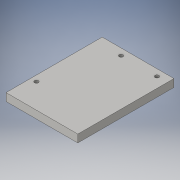
# Autodesk Inventor part: Arduino
Saved by Autodesk Inventor 2016 (Build 200138000, 138)
## iProperties
Created: 2018-09-29
Part Number: Arduino
Material: Generic
Document SubType Name: Modeling
Designer: Kyle
Density: 1 g/cm^3
Appearance: Default
Author: Kyle
## iProperties of the stored document Arduino_3DPrint.ipt
Created: 2018-09-30
Part Number: Arduino_3DPrint
Material: Generic
Document SubType Name: Modeling
Designer: Kyle
Density: 1 g/cm^3
Appearance: Default
Author: Kyle
Autodesk Inventor part; units mm, degrees
ref_plane "YZ Plane" through (0, 0, 0) normal (1, 0, 0) x (0, 1, 0)
ref_plane "XZ Plane" through (0, 0, 0) normal (0, 1, 0) x (-1, 0, 0)
ref_plane "XY Plane" through (0, 0, 0) normal (0, 0, 1) x (1, 0, 0)
sketch "Sketch1" plane through (0, 0, 0) normal (0, 1, 0) x (-1, 0, 0)
  circle A0 centre (24, 19) radius 1.5
  circle A1 centre (-19.5, -31.5) radius 1.5
  circle A2 centre (-19.5, -31.5) radius 1.5
  circle A3 centre (8.5, -31.5) radius 1.5
  line L0 (0, 0) -> (0, 17.5)
  line L1 (0, 17.5) -> (0, 19)
  line L2 (0, 19) -> (24, 19)
  line L3 (0, 0) -> (0, -31.5)
  line L4 (0, -31.5) -> (8.5, -31.5)
  line L5 (0, -31.5) -> (-19.5, -31.5)
  line L6 (0, 0) -> (2.25, 0)
  line L7 (-27.5, 38.25) -> (28.5, 38.25)
  line L8 (28.5, 38.25) -> (28.5, -36.75)
  line L9 (28.5, -36.75) -> (-27.5, -36.75)
  line L10 (-27.5, -36.75) -> (-27.5, 38.25)
  line L11 (-27.5, 38.25) -> (28.5, -36.75) construction
  line L12 (28.5, 38.25) -> (-27.5, -36.75) construction
  line L13 (-19.5, -31.5) -> (-19.5, -36.75)
  line L14 (25.5, 19) -> (28.5, 19)
  line L15 (28.5, 19) -> (28.5, -36.75)
  point P0 (0.5, 0.75)
  dimension "d2" = 3
  dimension "d0" = 3
  dimension "d1" = 3
  dimension "d3" = 17.5
  dimension "d4" = 8.5
  dimension "d5" = 19.5
  dimension "d6" = 31.5
  dimension "d7" = 24
  dimension "d12" = 43.5
  dimension "d13" = 2.25
  dimension "d14" = 56
  dimension "d15" = 75
  dimension "d16" = 5.25
  dimension "d17" = 3
  constraints: 32 end point, 6 horizontal, 5 vertical, 4 perpendicular, 3 centre point, 2 midpoint, 2 parallel, 2 point on line, 1 coincident, 1 concentric, 1 horizontal alignment, 3 other
  measures "d0" diameter of A3
  measures "d1" diameter of A1
  measures "d3" distance of L3.start L0.end
  measures "d4" distance of L4.start L4.end
  measures "d5" distance of L4.start L5.end
  measures "d6" distance of L3.start L4.start
  measures "d7" distance of L1.end L2.end
  measures "d12" horizontal distance of A1.centre L2.end
  measures "d13" distance of L6.start L6.end
  measures "d14" distance of L8.end L9.end
  measures "d15" distance of L8.end L7.end
  measures "d16" distance of L5.end L13.end
  measures "d17" distance of L14.start L14.end
extrude "Extrusion2" add sketch "Sketch1" along normal blind 6 contours L14 L8 L9 L13 A1 L5 L3 L0 L1 L2 A0 | A0 L2 L1 L0 L3 L5 A1 L13 L9 L10 L7 L8 L14
body "Solid2"
